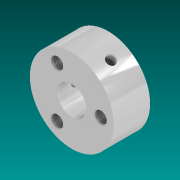
# Autodesk Inventor part: asmountAs4klein
Saved by Autodesk Inventor 2020.3 (Build 243373000, 373)
## iProperties
Created: 2020-05-24
Part Number: asmountAs4klein
Material: Aluminum 6061
Document SubType Name: Sheet Metal
Designer: Svend
Density: 2.7 g/cm^3
Sheet Metal Rule: Default_mm
Appearance: Aluminum - Polished
Flat Pattern Width: 2.3 cm
Flat Pattern Length: 2.3 cm
Flat Pattern Area: 5.29 cm^2
Sheet Metal Width: 23,000 mm
Sheet Metal Length: 23,000 mm
Sheet Metal Area: 529,000 mm^2
Author: Svend
Autodesk Inventor part; units mm, degrees
ref_plane "YZ Plane" through (0, 0, 0) normal (1, 0, 0) x (0, 1, 0)
ref_plane "XY Plane" through (0, 0, 0) normal (0, 0, 1) x (1, 0, 0)
sketch "Sketch1" plane through (0, 0, 0) normal (0, 0, 1) x (1, 0, 0)
  circle A0 centre (0, 0) radius 11.5
  circle A1 centre (0, 0) radius 4
  point P0 (8, 0)
  point P1 (-4, 6.9282)
  point P2 (-4, -6.9282)
  dimension "d0" = 23
  dimension "d1" = 8
  dimension "d2" = 8
  dimension "d5" = 360
  constraints: 2 centre point, 2 coincident, 1 horizontal alignment, 4 other
  measures "d0" diameter of A0
  measures "d1" distance of point (0, 0) point (8, 0)
  measures "d2" diameter of A1
extrude "Plate1" add sketch "Sketch1" along normal blind 10
hole "Hole1" at (8, 0, 0) at (-4, 6.9282, 0) at (-4, -6.9282, 0) direction (0, 0, 1) diameter 3.242 depth 15 tip angle 118 thread size "M4x0.7" class "6H" standard "ISO Metric profile"
sketch "Sketch2" plane through (0, 0, 0) normal (1, 0, 0) x (0, 1, 0)
  line L0 (4, 0) -> (-4, 0) projected
  point P0 (0, 0)
  point P1 (0, 5)
  dimension "d15" = 5
  constraints: 1 vertical alignment
  measures "d15" distance from line of L0 point (0, 5)
hole "Hole2" at (0, 0, 5) direction (-1, 0, 0) diameter 2.459 end through all thread size "M3x0.5" class "6H" standard "ISO Metric profile"
ref_plane "Work Plane1" through (0, 0, 0) normal (-0.5, -0.866, 0) x (0, 0, 1)
sketch "Sketch3" plane through (0, 0, 0) normal (-0.5, -0.866, 0) x (0, 0, 1)
  point P0 (0, 0)
  point P1 (5, 3.9111)
  point P2 (5, 0)
  dimension "d24" = 5
  constraints: 1 horizontal alignment, 1 other
  measures "d24" distance of point (5, 0) point (0, 0)
hole "Hole3" at (0, 0, 5) direction (0.5, 0.866, 0) diameter 2.459 end through all thread size "M3x0.5" class "6H" standard "ISO Metric profile"
equation "\"d7\" = Thickness"
equation "\"BendReliefDepth\" = 0.5 * Thickness"
equation "\"Thickness\" = 10"
body "Solid1"
